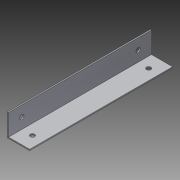
# Autodesk Inventor part: Hopper Bracing Front Right P7
Saved by Autodesk Inventor 2014 SP1 (Build 180222100, 222)
## iProperties
Created: 2013-12-16
Part Number: Hopper Bracing Front Right P7
Material: Aluminum 6061
Document SubType Name: Modeling
Designer: Moses
Mass: 6.6973 g
Surface Area: 64.6907 cm^2
Volume: 2.47133 cm^3
Density: 2.71 g/cm^3
Appearance: Aluminum - Flat
Author: Moses
Autodesk Inventor part; units mm, degrees
ref_plane "YZ Plane" through (0, 0, 0) normal (1, 0, 0) x (0, 1, 0)
ref_plane "XZ Plane" through (0, 0, 0) normal (0, 1, 0) x (-1, 0, 0)
ref_plane "XY Plane" through (0, 0, 0) normal (0, 0, 1) x (1, 0, 0)
sketch "Sketch1" plane through (0, 0, 0) normal (0, 0, 1) x (1, 0, 0)
  line L0 (0, 0) -> (0, 15.875)
  line L1 (0, 15.875) -> (0.7937, 15.875)
  line L2 (0.7937, 15.875) -> (0.7938, 0.7937)
  line L3 (0.7938, 0.7937) -> (15.875, 0.7937)
  line L4 (15.875, 0.7937) -> (15.875, 0)
  line L5 (15.875, 0) -> (0, 0)
  dimension "d0" = 15.875
  dimension "d1" = 0.7937
  constraints: 12 end point, 3 horizontal, 3 vertical, 2 perpendicular
  measures "d0" distance of L0.start L0.end
  measures "d1" distance of L0.end L1.end
extrude "Extrusion1" add sketch "Sketch1" along normal blind 101.6
sketch "Sketch2" plane through (0.7938, 0.7937, 0) normal (0, 1, 0) x (1, 0, 0)
  line L0 (0, 0) -> (15.0812, 0) projected
  line L1 (15.0812, -101.6) -> (0, -101.6) projected
  line L2 (7.5406, 0) -> (7.5406, -101.6) construction
  circle A0 centre (7.5406, -9.525) radius 1.5875
  circle A1 centre (7.5406, -92.075) radius 1.5875
  point P0 (-0.7938, 0)
  dimension "d4" = 9.525
  dimension "d5" = 3.175
  dimension "d6" = 101.6
  dimension "d9" = 82.55
  constraints: 2 centre point, 2 end point, 2 midpoint, 1 point on line, 1 vertical, 2 other
  measures "d4" distance from line of L0 A0.centre
  measures "d5" diameter of A0
  measures "d6" distance of L0.end L1.start
  measures "d9" distance of A0.centre A1.centre
sketch "Sketch3" plane through (0.7938, 0.7937, 0) normal (1, 0, 0) x (0, 0, -1)
  line L0 (0, 15.0812) -> (0, 0) projected
  line L1 (-101.6, 0) -> (-101.6, 15.0812) projected
  line L2 (-101.6, 7.5406) -> (0, 7.5406) construction
  circle A0 centre (-9.525, 7.5406) radius 1.5875
  circle A1 centre (-92.075, 7.5406) radius 1.5875
  point P0 (0, -0.7937)
  dimension "d14" = 3.175
  dimension "d15" = 9.525
  dimension "d16" = 101.6
  dimension "d19" = 82.55
  constraints: 2 centre point, 2 end point, 2 midpoint, 1 horizontal, 1 point on line, 2 other
  measures "d14" diameter of A0
  measures "d15" distance of L2.end A0.centre
  measures "d16" distance of L0.start L1.end
  measures "d19" distance of A0.centre A1.centre
extrude "Extrusion2" cut sketch "Sketch2" against normal through all
extrude "Extrusion3" cut sketch "Sketch3" against normal through all
body "Solid1"
